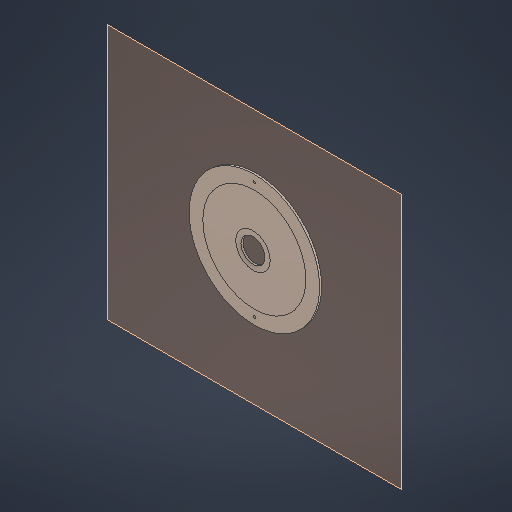
# Autodesk Inventor part: Prressure plate
Saved by Autodesk Inventor 2026.3 (Build 303398000, 398)
## iProperties
Created: 2026-07-26
Part Number: Prressure plate
Material: Generic
Document SubType Name: Sheet Metal
Designer: matot
Density: 1 g/cm^3
Sheet Metal Rule: Default_mm
Appearance: Default
Author: matot
Autodesk Inventor part; units mm, degrees
ref_plane "YZ Plane" through (0, 0, 0) normal (1, 0, 0) x (0, 1, 0)
ref_plane "XZ Plane" through (0, 0, 0) normal (0, 1, 0) x (-1, 0, 0)
ref_plane "XY Plane" through (0, 0, 0) normal (0, 0, 1) x (1, 0, 0)
sketch "Sketch1" plane through (0, 0, 0) normal (1, 0, 0) x (0, 1, 0)
  line L0 (0, 0) -> (95, 0)
  line L1 (95, 0) -> (95, 3)
  line L2 (0, 3) -> (0, 0)
  line L3 (0, 0) -> (38.25, 0)
  line L4 (25, 5) -> (0, 5)
  line L5 (0, 5) -> (0, 0)
  line L6 (0, 5) -> (25, 5)
  line L7 (25, 3) -> (25, 2)
  line L8 (25, 2) -> (0, 2)
  line L9 (0, 2) -> (0, 5)
  line L10 (95, 3) -> (75, 3)
  line L11 (75, 0) -> (95, 0)
  line L12 (95, 0) -> (95, 3)
  line L13 (75, 0) -> (25, 2)
  line L14 (75, 3) -> (25, 5)
  point P0 (0, 3.5)
  point P1 (25, 3.5)
  point P2 (0, 2)
  point P3 (95, 1.5)
  dimension "d2" = 5
  dimension "d3" = 25
  dimension "d4" = 3
  dimension "d5" = 3
  dimension "d6" = 25
  dimension "d52" = 50
  dimension "d53" = 50
  dimension "d54" = 20
  constraints: 30 end point, 5 parallel, 4 horizontal, 3 point on line, 2 midpoint, 2 perpendicular
  measures "d2" distance of L0.start L4.end
  measures "d3" distance of L4.start L4.end
  measures "d4" distance of L6.end L7.end
  measures "d5" distance of L0.end L1.end
  measures "d6" distance of point (0, 3.5) point (25, 3.5)
  measures "d52" horizontal distance of L11.start L7.end
  measures "d53" horizontal distance of L4.start L10.end
  measures "d54" horizontal distance of L10.end point (95, 1.5)
revolve "Revolution1" add sketch "Sketch1" angle 360 about axis through (0, 0, 5) along (0, 0, -1) contours L2 L5 L4 L14 L10 L1 L0 L13 L8
sketch "Sketch2" plane through (0, 0, 5) normal (0, 0, 1) x (1, 0, 0)
  circle A0 centre (0, 0) radius 17.5
  dimension "d9" = 35
  constraints: 1 centre point, 1 coincident
  measures "d9" diameter of A0
extrude "Extrusion1" cut sketch "Sketch2" against normal through all
ref_plane "Work Plane1" through (0, 0, 5) normal (0, 0, 1) x (1, 0, 0)
sketch "Sketch6" plane through (0, 0, 3) normal (0, 0, 1) x (1, 0, 0)
  point P0 (0, 0)
  point P1 (0, 85)
  point P2 (0, -85)
  dimension "d86" = 85
  dimension "d87" = 85
  measures "d86" distance of point (0, 0) point (0, -85)
  measures "d87" distance of point (0, 0) point (0, 85)
hole "Hole1" at (0, 85, 3) at (0, -85, 3) direction (0, 0, -1) diameter 3.4587 end through all thread size "M4x0.5" class "6H" standard "ISO Metric profile"
equation "\"d93\" = Thickness"
equation "\"BendRadius\" = Thickness"
equation "\"BendReliefWidth\" = Thickness"
equation "\"BendReliefDepth\" = 0.5 * Thickness"
equation "\"CornerReliefSize\" = 4 * Thickness"
equation "\"MinimumRemnant\" = 2 * Thickness"
equation "\"TransitionRadius\" = BendRadius"
equation "\"JacobiRadiusSize\" = BendRadius"
equation "\"GapSize\" = Thickness"
equation "\"Thickness\" = 0.5"
body "Solid1"
